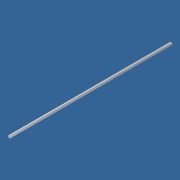
# Autodesk Inventor part: GE-12056
Saved by Autodesk Inventor 2012 (Build 160160000, 160)
## iProperties
Created: 2010-11-10
Part Number: GE-12056
Document SubType Name: Modeling
Designer: mcyr
Density: 1 g/cm^3
Description: Inner Tube
Material: Default
Title: Inner Tube
Author: mcyr
Autodesk Inventor part; units mm, degrees
ref_plane "YZ Plane" through (0, 0, 0) normal (1, 0, 0) x (0, 1, 0)
ref_plane "XY Plane" through (0, 0, 0) normal (0, 0, 1) x (1, 0, 0)
sketch "Sketch1" plane through (0, 0, 0) normal (0, 0, 1) x (1, 0, 0)
  circle A0 centre (0, 0) radius 13.208
  circle A1 centre (0, 0) radius 16.637
  dimension "d0" = 33.274
  dimension "d1" = 26.416
  constraints: 2 centre point, 2 coincident
  measures "d0" diameter of A1
  measures "d1" diameter of A0
extrude "Extrusion1" add sketch "Sketch1" along normal blind 2082.8
ref_plane "Work Plane1" through (0, 0, 2082.8) normal (0, 1, 0) x (0, 0, -1)
sketch "Sketch2" plane through (0, 0, 0) normal (0, 1, 0) x (-1, 0, 0)
  line L0 (-16.637, 2082.8) -> (16.637, 2082.8) projected
  line L1 (16.637, 2082.8) -> (16.637, 0) projected
  line L2 (16.637, 0) -> (13.208, 0) projected
  line L3 (13.208, 0) -> (13.208, 2082.8) projected
  line L4 (13.208, 2082.8) -> (16.637, 2082.8) projected
  line L5 (-16.637, 0) -> (-16.637, 2082.8) projected
  line L6 (-16.637, 2082.8) -> (-13.208, 2082.8) projected
  line L7 (-13.208, 2082.8) -> (-13.208, 0) projected
  line L8 (-13.208, 0) -> (-16.637, 0) projected
  line L9 (13.208, 0) -> (-13.208, 0) projected
  circle A0 centre (0, 34.9504) radius 3.9688
  point P0 (0, 0)
  dimension "d13" = 7.9375
  constraints: 1 centre point
  measures "d13" diameter of A0
extrude "Extrusion2" cut sketch "Sketch2" against normal mid plane 35.56 contours A0
body "Solid1"
